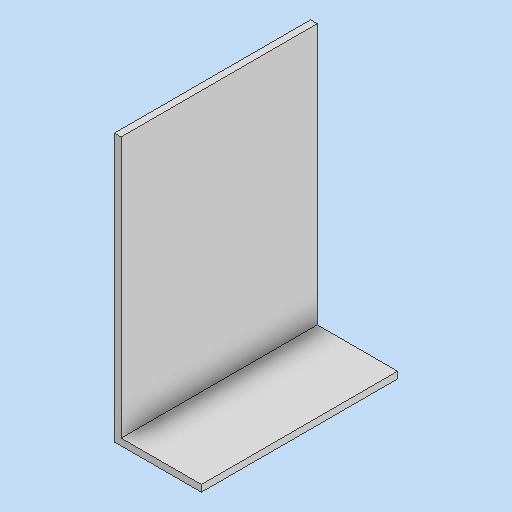
# Autodesk Inventor part: inside walls front
Saved by Autodesk Inventor 2026 (Build 300175000, 175)
## iProperties
Created: 2026-02-03
Part Number: inside walls front
Material: Generic
Document SubType Name: Modeling
Designer: mones
Density: 1 g/cm^3
Appearance: Default
Author: mones
Autodesk Inventor part; units mm, degrees
ref_plane "YZ Plane" through (0, 0, 0) normal (1, 0, 0) x (0, 1, 0)
ref_plane "XZ Plane" through (0, 0, 0) normal (0, 1, 0) x (-1, 0, 0)
ref_plane "XY Plane" through (0, 0, 0) normal (0, 0, 1) x (1, 0, 0)
sketch "Sketch1" plane through (0, 0, 0) normal (1, 0, 0) x (0, 1, 0)
  line L0 (98.5, 44) -> (98.5, -44)
  line L1 (98.5, -44) -> (-21.5, -44)
  line L2 (-21.5, -44) -> (-21.5, 44)
  line L3 (-21.5, 44) -> (98.5, 44)
  line L4 (98.5, 44) -> (-21.5, -44) construction
  line L5 (98.5, -44) -> (-21.5, 44) construction
  point P0 (38.5, 0)
  dimension "d0" = 88
  dimension "d1" = 120
  constraints: 12 end point, 2 midpoint, 2 parallel, 1 perpendicular, 1 vertical
  measures "d0" distance of L0.start L0.end
  measures "d1" distance of L0.end L1.end
extrude "Extrusion1" add sketch "Sketch1" along normal blind 3
sketch "Sketch2" plane through (3, 0, 0) normal (1, 0, 0) x (0, 0, -1)
  line L0 (-44, -21.5) -> (44, -21.5) projected
  line L1 (44, -21.5) -> (44, 98.5) projected
  line L2 (44, 98.5) -> (-44, 98.5) projected
  line L3 (-44, 98.5) -> (-44, -21.5) projected
  line L4 (44, -21.5) -> (-44, -21.5)
  line L5 (-44, -21.5) -> (-44, -18.5)
  line L6 (-44, -18.5) -> (44, -18.5)
  line L7 (44, -18.5) -> (44, -21.5)
  dimension "d4" = 3
  constraints: 8 end point, 2 perpendicular, 2 point on line, 1 horizontal
  measures "d4" distance of L0.start L5.end
extrude "Extrusion2" add sketch "Sketch2" along normal blind 36 contours L3 L6 L1 L0
body "Solid1"
